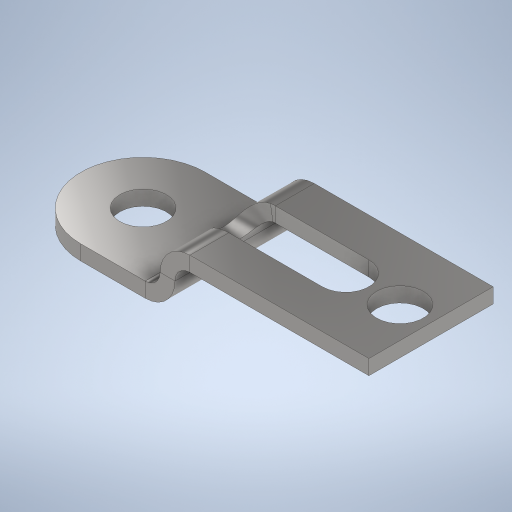
# Autodesk Inventor part: BoxMountingMetal
Saved by Autodesk Inventor 2024.2 (Build 282272000, 272)
## iProperties
Created: 2024-01-23
Part Number: BoxMountingMetal
Material: Stainless Steel, Austenitic
Document SubType Name: Sheet Metal
Designer: airso
Density: 8 g/cm^3
Sheet Metal Rule: Default
Appearance: Semi-Polished
Author: airso
Autodesk Inventor part; units mm, degrees
ref_plane "YZ Plane" through (0, 0, 0) normal (1, 0, 0) x (0, 1, 0)
ref_plane "XZ Plane" through (0, 0, 0) normal (0, 1, 0) x (-1, 0, 0)
ref_plane "XY Plane" through (0, 0, 0) normal (0, 0, 1) x (1, 0, 0)
sketch "Sketch1" plane through (0, 0, 0) normal (0, 1, 0) x (-1, 0, 0)
  circle A0 centre (0, 0) radius 6.35
  circle A1 centre (0, 0) radius 2.3813
  line L0 (0, 6.35) -> (-31.75, 6.35)
  line L1 (-31.75, 6.35) -> (-31.75, -6.35)
  line L2 (-31.75, -6.35) -> (0, -6.35)
  line L3 (0, -6.35) -> (0, 6.35)
  circle A2 centre (-28.575, 0) radius 2.3813
  line L4 (-13.0948, 2.3812) -> (-23.0187, 2.3812)
  line L5 (-13.0948, -2.3813) -> (-23.0187, -2.3813)
  arc A3 (-13.0948, -2.3813) -> (-13.0948, 2.3812) centre (-13.0948, 0) ccw
  arc A4 (-23.0187, 2.3812) -> (-23.0187, -2.3813) centre (-23.0187, 0) ccw
  point P0 (-31.75, 0)
  dimension "d0" = 12.7
  dimension "d1" = 4.7625
  dimension "d2" = 31.75
  dimension "d3" = 12.7
  dimension "d4" = 4.7625
  dimension "d5" = 3.175
  dimension "d6" = 6.35
  dimension "d7" = 2.3813
  dimension "d8" = 3.9688
  dimension "d9" = 5.5563
  measures "d1" diameter of A1
  measures "d2" distance of L1.end L2.end
  measures "d3" distance of L0.end L1.end
  measures "d4" diameter of A2
  measures "d5" distance of point (-31.75, 0) A2.centre
  measures "d6" distance from line of L0 A2.centre
  measures "d7" radius of A3
  measures "d8" distance between parallel lines of L0 L4
  measures "d9" distance of A2.centre A4.centre
extrude "Plate1" add sketch "Sketch1" along normal blind 1.524 contours A0 L3 A1 | L3 A1 A0 | A0 L2 L1 L0
sketch "Sketch2" plane through (0, 1.524, 0) normal (0, 1, 0) x (1, 0, 0)
  line L0 (0, -6.35) -> (31.75, -6.35) projected
  line L1 (13.462, -6.35) -> (13.462, 6.35)
  line L2 (31.75, 6.35) -> (0, 6.35) projected
  line L3 (31.75, 6.35) -> (31.75, -6.35) projected
  line L4 (6.3638, -6.35) -> (6.3638, 6.35)
  arc A0 (13.0948, 2.3813) -> (13.0948, -2.3812) centre (13.0948, 0) ccw projected
  point P0 (0, 0)
  point P1 (10.7136, 0)
  dimension "d11" = 18.288
  dimension "d13" = 6.731
  constraints: 4 end point, 4 point on line, 1 perpendicular, 1 point on circle, 1 vertical
  measures "d11" distance between parallel lines of L3 L1
  measures "d13" distance from line of A0.centre L4
fold "Fold1" angle 90 bend radius 1.524 thickness 1.524 k factor 0.44 line from (13.462, 1.524, 6.35) to (13.462, 1.524, -6.35) line at bend start moving side (-1, 0, 0) folds toward (0, -1, 0)
sketch "Sketch3" plane through (10.414, -11.5388, -6.35) normal (-1, 0, 0) x (0, 0, 1)
  line L0 (0, 10.0148) -> (12.7, 10.0148) projected
  line L1 (0, 10.0148) -> (12.7, 10.0148)
  point P0 (6.35, 11.5388)
  constraints: 2 end point, 1 collinear
fold "Fold2" angle 90 bend radius 1.524 thickness 1.524 k factor 0.44 line from (10.414, -1.524, -6.35) to (10.414, -1.524, 6.35) line at bend start moving side (0, -1, 0) folds toward (-1, 0, 0)
equation "\"d10\" = Thickness"
equation "\"d14\" = BendReliefWidth"
equation "\"d15\" = BendReliefDepth"
equation "\"d16\" = MinimumRemnant"
equation "\"d17\" = TransitionRadius"
equation "\"d19\" = BendRadius"
equation "\"d20\" = BendReliefWidth"
equation "\"d21\" = BendReliefDepth"
equation "\"d22\" = MinimumRemnant"
equation "\"d23\" = TransitionRadius"
equation "\"d25\" = BendRadius"
equation "\"BendRadius\" = Thickness"
equation "\"BendReliefWidth\" = Thickness"
equation "\"BendReliefDepth\" = 0.5 * Thickness"
equation "\"CornerReliefSize\" = 4 * Thickness"
equation "\"MinimumRemnant\" = 2 * Thickness"
equation "\"TransitionRadius\" = BendRadius"
equation "\"JacobiRadiusSize\" = BendRadius"
equation "\"GapSize\" = Thickness"
equation "\"Thickness\" = 1.524"
body "Solid1"
